A4 (Autodesk Fusion 360 design; units mm, degrees)
Autodesk Fusion 360 part; units mm, degrees
sketch "Sketch" plane through (0, 0, 0) normal (0, 0, 1) x (-1, 0, 0)
  line L0 (0, 80) -> (0, 0)
  line L1 (-40, 0) -> (-40, 80)
  line L2 (0, 0) -> (-40, 0)
  line L3 (-40, 80) -> (0, 80)
  line L4 (0, 0) -> (0, 20)
  line L5 (0, 60) -> (0, 20)
  line L6 (-40, 20) -> (-40, 60)
  line L7 (0, 20) -> (-40, 20)
  line L8 (-40, 60) -> (0, 60)
  line L9 (-20, 0) -> (0, 0) construction
  arc A0 (-40, 0) -> (0, 0) centre (-20, 0) ccw
  line L10 (-20, 0) -> (-40, 0) construction
  line L11 (-20, 80) -> (-40, 80) construction
  arc A1 (0, 80) -> (-40, 80) centre (-20, 80) ccw
  line L12 (-20, 80) -> (0, 80) construction
  circle A2 centre (-20, 0) radius 10
  circle A3 centre (-20, 80) radius 10
  dimension "d2" = 40
  dimension "d3" = 20
  dimension "d4" = 40
  dimension "d5" = 20
  dimension "d8" = 20
  dimension "d9" = 20
  constraint vertical L0
  constraint vertical L1
  constraint coincident L0.end L2.start
  constraint horizontal L3
  constraint horizontal L2
  constraint coincident L0 L4.end
  constraint vertical L5
  constraint vertical L6
  constraint horizontal L8
  constraint horizontal L7
  constraint midpoint L2 L9.start
  constraint coincident L9.start A0.centre
  constraint coincident L0.start L3.end
  constraint midpoint L3 L11.start
  constraint coincident L11.start A1.centre
  constraint concentric A0 A2
  constraint concentric A1 A3
  measures "d2" distance of L0.end L1.start
  measures "d3" distance of L0.end L4.end
  measures "d4" distance of L4.end L5.start
  measures "d5" distance of L0.start L5.start
  measures "d8" diameter of A2
  measures "d9" diameter of A3
extrude "Extrude1" add sketch "Sketch" along normal blind 10 contours L0 L1 L3 L8 A3 | L3 A1 A3 | L0 L1 L5 L6 L7 L8 | L0 L1 L2 L4 L7 A2 | L2 A0 A2
sketch "Sketch 1" plane through (0, 0, 0) normal (1, 0, 0) x (0, 1, 0)
  line L0 (0, 0) -> (-20, 0)
  line L1 (-20, 10) -> (0, 10)
  line L2 (-20, 0) -> (-20, 10)
  line L3 (0, 10) -> (0, 0)
  line L4 (-20, 10) -> (-20, 0)
  line L5 (-60, 10) -> (-20, 10)
  line L6 (-20, 0) -> (-60, 0)
  line L7 (-60, 0) -> (-60, 10)
  line L8 (-60, 10) -> (-60, 0)
  line L9 (-80, 10) -> (-60, 10)
  line L10 (-60, 0) -> (-80, 0)
  line L11 (-80, 0) -> (-80, 10)
  line L12 (-60, 10) -> (-60, 30)
  line L13 (-20, 10) -> (-60, 10)
  line L14 (-60, 30) -> (-20, 30)
  line L15 (-20, 30) -> (-20, 10)
  line L16 (-40, 30) -> (-60, 30) construction
  line L17 (-40, 30) -> (-20, 30) construction
  arc A0 (-20, 30) -> (-60, 30) centre (-40, 30) ccw
  circle A1 centre (-40, 30) radius 10
  dimension "d13" = 20
  constraint horizontal L0
  constraint coincident L0.start L3.end
  constraint horizontal L1
  constraint vertical L2
  constraint vertical L3
  constraint horizontal L5
  constraint horizontal L6
  constraint vertical L4
  constraint vertical L7
  constraint horizontal L9
  constraint vertical L8
  constraint horizontal L10
  constraint vertical L11
  constraint vertical L12
  constraint horizontal L14
  constraint vertical L15
  constraint horizontal L13
  constraint coincident L14.end L15.start
  constraint midpoint L14 L16.start
  constraint coincident L16.start L17.start
  constraint concentric A0 A1
  measures "d13" diameter of A1
extrude "Extrude2" add sketch "Sketch 1" along normal blind 40 contours L2 L4 L5 L6 L7 L8 L13 | L5 L12 L13 L14 L15 A1 | L14 A0 A1
